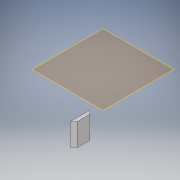
# Autodesk Inventor part: last_drill_slide_fit
Saved by Autodesk Inventor 2019 (Build 230136000, 136)
## iProperties
Created: 2018-12-20
Part Number: last_drill_slide_fit
Material: Generic
Document SubType Name: Modeling
Designer: assman
Density: 1 g/cm^3
Appearance: Default
Author: assman
## iProperties of the stored document last_drill_slide_fit_3DPrint.ipt
Created: 2018-12-20
Part Number: last_drill_slide_fit_3DPrint
Material: Generic
Document SubType Name: Modeling
Designer: assman
Density: 1 g/cm^3
Appearance: Default
Author: assman
Autodesk Inventor part; units mm, degrees
ref_plane "YZ Plane" through (0, 0, 0) normal (1, 0, 0) x (0, 1, 0)
ref_plane "XZ Plane" through (0, 0, 0) normal (0, 1, 0) x (-1, 0, 0)
ref_plane "XY Plane" through (0, 0, 0) normal (0, 0, 1) x (1, 0, 0)
ref_plane "Work Plane1" through (-10, 7, -20) normal (0, 1, 0) x (1, 0, 0)
sketch "Sketch3" plane through (-10, 7, -20) normal (0, 1, 0) x (1, 0, 0)
  line L0 (8.9293, -13.0418) -> (10, -14.1125) projected
  line L1 (8.9293, -19.0438) -> (8.9293, -13.0418) projected
  line L2 (10, -17.9731) -> (8.9293, -19.0438) projected
  line L3 (8.9293, -19.0438) -> (10, -17.9731) projected
  line L4 (10, -17.9731) -> (8.9293, -19.0438)
  line L5 (8.9293, -13.0418) -> (8.9293, -19.0438) projected
  line L6 (8.9293, -19.0438) -> (8.9293, -13.0418)
  line L7 (8.9293, -13.0418) -> (10, -14.1125)
  line L8 (10, -14.1125) -> (10, -17.9731)
  line L9 (10, -14.1125) -> (8.9293, -13.0418) projected
  line L10 (10, -17.9731) -> (10, -14.1125)
  line L11 (10, -14.1125) -> (10, -17.9731)
  point P0 (10, -20)
  constraints: 12 end point, 4 collinear, 1 vertical
extrude "Extrusion1" add sketch "Sketch3" against normal blind 7
body "Solid2"
body "Solid1"
